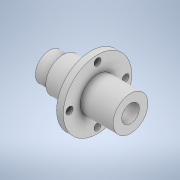
# Autodesk Inventor part: pilot
Saved by Autodesk Inventor 2020 (Build 240168000, 168)
## iProperties
Created: 2020-03-12
Part Number: pilot
Material: Generic
Document SubType Name: Modeling
Designer: jgranlund
Density: 1 g/cm^3
Appearance: Default
Author: jgranlund
Autodesk Inventor part; units mm, degrees
ref_plane "YZ Plane" through (0, 0, 0) normal (1, 0, 0) x (0, 1, 0)
ref_plane "XZ Plane" through (0, 0, 0) normal (0, 1, 0) x (-1, 0, 0)
ref_plane "XY Plane" through (0, 0, 0) normal (0, 0, 1) x (1, 0, 0)
sketch "Sketch1" plane through (0, 0, 0) normal (0, 0, 1) x (1, 0, 0)
  line L0 (0, 0) -> (0, 31.5)
  line L1 (0, 31.5) -> (-60, 31.5)
  line L2 (-60, 31.5) -> (-60, 62)
  line L3 (-60, 62) -> (-72, 62)
  line L4 (-72, 62) -> (-72, 31.5)
  line L5 (-72, 31.5) -> (-122, 31.5)
  line L6 (-122, 31.5) -> (-122, 25.5)
  line L7 (-122, 25.5) -> (-147, 25.5)
  line L8 (-147, 25.5) -> (-147, 0)
  line L9 (-147, 0) -> (0, 0)
  dimension "d0" = 31.5
  dimension "d1" = 60
  dimension "d2" = 30.5
  dimension "d3" = 12
  dimension "d4" = 30.5
  dimension "d5" = 50
  dimension "d6" = 6
  dimension "d7" = 25
  constraints: 20 end point, 6 perpendicular, 2 point on line, 1 horizontal, 1 vertical
  measures "d0" distance of L0.start L0.end
  measures "d1" distance of L0.end L1.end
  measures "d2" distance of L1.end L2.end
  measures "d3" distance of L2.end L3.end
  measures "d4" distance of L3.end L4.end
  measures "d5" distance of L4.end L5.end
  measures "d6" distance of L5.end L6.end
  measures "d7" distance of L6.end L7.end
revolve "Revolution1" add sketch "Sketch1" angle 360 about axis through (-147, 0, 0) along (1, 0, 0)
sketch "Sketch2" plane through (-60, 0, 0) normal (1, 0, 0) x (0, 0, -1)
  circle A0 centre (0, 50.8) radius 6.35
  circle A1 centre (-50.8, 0) radius 6.35
  circle A2 centre (50.8, 0) radius 6.35
  circle A3 centre (0, -50.8) radius 6.35
  line L0 (0, 0) -> (0, 50.8) construction
  line L1 (0, 0) -> (0, 50.8) construction
  line L2 (0, 0) -> (50.8, 0) construction
  line L3 (0, 0) -> (0, -50.8) construction
  line L4 (0, 0) -> (-50.8, 0) construction
  dimension "d9" = 12.7
  dimension "d10" = 50.8
  dimension "d11" = 12.7
  dimension "d12" = 12.7
  dimension "d13" = 12.7
  constraints: 10 end point, 4 centre point, 3 equal length, 2 horizontal, 2 vertical, 1 collinear
  measures "d9" diameter of A0
  measures "d10" distance of L0.end L0.start
  measures "d11" diameter of A1
  measures "d12" diameter of A2
  measures "d13" diameter of A3
extrude "Extrusion1" cut sketch "Sketch2" against normal through all
sketch "Sketch3" plane through (0, 0, 0) normal (1, 0, 0) x (0, 0, -1)
  circle A0 centre (0, 0) radius 16
  dimension "d16" = 32
  constraints: 1 centre point, 1 coincident
  measures "d16" diameter of A0
extrude "Extrusion2" cut sketch "Sketch3" against normal blind 60
body "Solid1"
